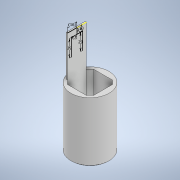
# Autodesk Inventor part: brazo_base_2
Saved by Autodesk Inventor 2021 (Build 250183000, 183)
## iProperties
Created: 2021-03-16
Part Number: brazo_base_2
Material: Genérico
Document SubType Name: Modeling
Designer: Joaquín
Density: 1 g/cm^3
Appearance: Valor por defecto
Author: Joaquín
Autodesk Inventor part; units mm, degrees
ref_plane "YZ Plane" through (0, 0, 0) normal (1, 0, 0) x (0, 1, 0)
ref_plane "XZ Plane" through (0, 0, 0) normal (0, 1, 0) x (-1, 0, 0)
ref_plane "XY Plane" through (0, 0, 0) normal (0, 0, 1) x (1, 0, 0)
sketch "Boceto1" plane through (0, 0, 0) normal (0, 1, 0) x (-1, 0, 0)
  circle A0 centre (0, 0) radius 32.5
  line L0 (0, 22.5) -> (16, 22.5)
  line L1 (0, 0) -> (22.5, 0)
  line L2 (22.5, 0) -> (22.5, 16)
  line L3 (22.5, 16) -> (16, 22.5)
  line L4 (0, 22.5) -> (-16, 22.5)
  line L5 (-16, 22.5) -> (-22.5, 16)
  line L6 (-22.5, 0) -> (-22.5, 16)
  line L7 (-22.5, 0) -> (-22.5, -16)
  line L8 (-22.5, -16) -> (-16, -22.5)
  line L9 (0, -22.5) -> (-16, -22.5)
  line L10 (0, -22.5) -> (16, -22.5)
  line L11 (16, -22.5) -> (22.5, -16)
  line L12 (22.5, 0) -> (22.5, -16)
  dimension "d3" = 22.5
  dimension "d7" = 360
  constraints: 26 end point, 1 centre point, 1 coincident, 1 horizontal, 1 perpendicular, 29 other
  measures "d3" distance of L1.start L1.end
extrude "Extrusión1" add sketch "Boceto1" along normal blind 100
sketch "Boceto2" plane through (0, 0, 0) normal (0, -1, 0) x (1, 0, 0)
  circle A0 centre (0, 0) radius 29.8
  circle A1 centre (0, 0) radius 30.25
  dimension "d11" = 59.6
  dimension "d12" = 60.5
  constraints: 2 centre point, 2 coincident
  measures "d11" diameter of A0
  measures "d12" diameter of A1
extrude "Extrusión2" add sketch "Boceto2" along normal blind 2
sketch "Boceto6" plane through (0, 100, 0) normal (0, 1, 0) x (1, 0, 0)
  line L0 (-22.5, -16) -> (-22.5, 16) projected
  line L1 (-22.5, -16) -> (-22.5, 16)
  line L2 (-22.5, 16) -> (-24.5, 16)
  line L3 (-24.5, 16) -> (-24.5, -16)
  line L4 (-24.5, -16) -> (-22.5, -16)
  point P0 (0, 0)
  dimension "d38" = 2
  constraints: 8 end point, 3 perpendicular, 1 collinear
  measures "d38" distance of L0.end L2.end
extrude "Extrusión4" add sketch "Boceto6" along normal blind 70
sketch "Boceto7" plane through (-22.5, 0, 16) normal (1, 0, 0) x (0, 0, -1)
  line L0 (0, 170) -> (32, 170) projected
  line L1 (0, 170) -> (16, 170)
  line L2 (16, 170) -> (16, 160)
  line L3 (16, 160) -> (6.5, 160)
  line L4 (16, 160) -> (25.5, 160)
  line L5 (6.5, 160) -> (6.5, 131)
  line L6 (25.5, 160) -> (25.5, 131)
  point P0 (16, 0)
  dimension "d41" = 16
  dimension "d42" = 10
  dimension "d43" = 9.5
  dimension "d44" = 9.5
  dimension "d45" = 29
  dimension "d46" = 29
  constraints: 12 end point, 2 vertical, 1 horizontal, 1 midpoint, 1 parallel, 1 perpendicular
  measures "d41" distance of L0.start L1.end
  measures "d42" distance of L1.end L2.end
  measures "d43" distance of L2.end L3.end
  measures "d44" distance of L2.end L4.end
  measures "d45" distance of L3.end L5.end
  measures "d46" distance of L4.end L6.end
